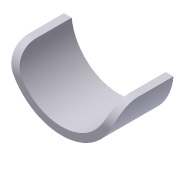
# Autodesk Inventor part: FE-00006-08
Saved by Autodesk Inventor 2012 (Build 160160000, 160)
## iProperties
Created: 2008-05-25
Part Number: FE-00006-08
Document SubType Name: Modeling
Designer: firstuser
Density: 1 g/cm^3
Mass: 5.67768 g
Surface Area: 39.2817 cm^2
Volume: 5.67768 cm^3
Material: Default
Author: firstuser
Autodesk Inventor part; units mm, degrees
ref_plane "YZ Plane" through (0, 0, 0) normal (1, 0, 0) x (0, 1, 0)
ref_plane "XZ Plane" through (0, 0, 0) normal (0, 1, 0) x (-1, 0, 0)
ref_plane "XY Plane" through (0, 0, 0) normal (0, 0, 1) x (1, 0, 0)
sketch "Sketch1" plane through (0, 0, 0) normal (0, 0, 1) x (1, 0, 0)
  arc A0 (-73.7988, 68.3559) -> (-25.1062, 68.3559) centre (-49.4525, 70.5784) ccw
  arc A1 (-70.366, 68.3559) -> (-28.5391, 68.3559) centre (-49.4525, 70.5784) ccw
  line L0 (-73.7988, 68.3559) -> (-70.366, 68.3559)
  line L1 (-28.5391, 68.3559) -> (-25.1062, 68.3559)
  dimension "d0" = 22.225
  dimension "d1" = 21.0312
  dimension "d2" = 24.4475
  constraints: 4 end point, 4 point on circle, 2 centre point, 2 collinear, 1 concentric, 1 horizontal
  measures "d0" distance edge to line of A0 L0
  measures "d1" radius of A1
  measures "d2" radius of A0
extrude "Extrusion1" add sketch "Sketch1" along normal blind 25.4
fillet "Fillet1" radius 9.525 2 edges at (-72.0824, 68.3559, 25.4) (-26.8227, 68.3559, 25.4)
body "Solid1"
